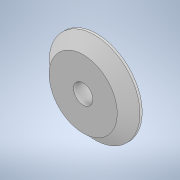
# Autodesk Inventor part: plastic_wheel_washer
Saved by Autodesk Inventor 2020 (Build 240168000, 168)
## iProperties
Created: 2019-08-05
Part Number: plastic_wheel_washer
Material: Generic
Document SubType Name: Modeling
Designer: erwin
Density: 1 g/cm^3
Appearance: Default
Author: erwin
Autodesk Inventor part; units mm, degrees
ref_plane "YZ Plane" through (0, 0, 0) normal (1, 0, 0) x (0, 1, 0)
ref_plane "XZ Plane" through (0, 0, 0) normal (0, 1, 0) x (-1, 0, 0)
ref_plane "Work Plane1" through (0, 0, 0) normal (0, 0, 1) x (1, 0, 0)
sketch "Sketch1" plane through (0, 0, 0) normal (0, 0, 1) x (1, 0, 0)
  arc A0 (63.0305, 195.3497) -> (48.9551, 209.4251) centre (68.2595, 214.6541) ccw
  circle A1 centre (68.2595, 214.6541) radius 4.25
  circle A2 centre (68.2595, 214.6541) radius 20
  point P0 (0, 0)
  point P1 (28.2595, 174.6541)
  dimension "d1" = 40
  dimension "d2" = 8.5
  constraints: 3 centre point, 3 coincident, 2 point on circle, 1 concentric
  measures "d1" diameter of A0
  measures "d2" diameter of A1
extrude "Extrusion1" add sketch "Sketch1" along normal blind 6
chamfer "Chamfer1" distance 5 angle 45 1 edges at (82.4016, 228.7962, 6)
body "Solid1"
